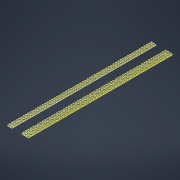
# Autodesk Inventor part: 110033226_ipt_39_背流基座
Saved by Autodesk Inventor 2022 (Build 260153000, 153)
## iProperties
Created: 2022-06-26
Part Number: 110033226_ipt_39_背流基座
Material: 一般
Document SubType Name: Modeling
Designer: User
Density: 1 g/cm^3
Appearance: 預設
Author: User
Autodesk Inventor part; units mm, degrees
ref_plane "YZ Plane" through (0, 0, 0) normal (1, 0, 0) x (0, 1, 0)
ref_plane "XZ Plane" through (0, 0, 0) normal (0, 1, 0) x (-1, 0, 0)
ref_plane "XY Plane" through (0, 0, 0) normal (0, 0, 1) x (1, 0, 0)
sketch "草圖1" plane through (0, 0, 0) normal (0, 1, 0) x (-1, 0, 0)
  line L0 (0, 0) -> (40, 0)
  line L1 (40, 0) -> (40, -305)
  line L2 (40, -305) -> (0, -305)
  line L3 (0, -305) -> (0, 0)
  circle A0 centre (2.5, -2.5) radius 1.7
  line L4 (10, -305) -> (10, 0)
  line L5 (30, -305) -> (30, 0)
  dimension "d0" = 40
  dimension "d1" = 305
  dimension "d2" = 3.4
  dimension "d3" = 2.5
  dimension "d4" = 2.5
  dimension "d45" = 10
  dimension "d46" = 10
  constraints: 12 end point, 4 point on line, 3 perpendicular, 2 parallel, 1 centre point, 1 horizontal
  measures "d0" distance of L1.end L2.end
  measures "d1" distance of L0.end L1.end
  measures "d2" diameter of A0
  measures "d3" distance from line of L3 A0.centre
  measures "d4" distance from line of L0 A0.centre
  measures "d45" distance between parallel lines of L3 L4
  measures "d46" distance between parallel lines of L1 L5
extrude "擠出1" add sketch "草圖1" along normal blind 2.5 contours L0 L4 L2 L3 | L0 L1 L2 L5 | A0
extrude "擠出2" cut sketch "草圖1" along normal blind 1.5 contours A0
sketch "草圖2" plane through (0, 2.5, 0) normal (0, 1, 0) x (1, 0, 0)
  circle A0 centre (-2.5, 2.5) radius 1.7 projected
  point P0 (0, 0)
extrude "擠出3" add sketch "草圖2" along normal blind 1.5
pattern_linear "矩形陣列3" count 61 spacing 5 along (0, 0, -1) count 2 spacing 5 along (-1, 0, 0) of "擠出3", "擠出2"
sketch "草圖3" plane through (0, 2.5, 0) normal (0, 1, 0) x (1, 0, 0)
  circle A0 centre (-2.5, 2.5) radius 1.7 projected
  line L0 (0, 305) -> (0, 0) projected
  line L1 (-30, 0) -> (-40, 0) projected
  line L2 (-40, 0) -> (-40, 305) projected
  line L3 (-40, 305) -> (-30, 305) projected
  circle A1 centre (-2.5, 7.5) radius 1.7 projected
  circle A2 centre (-2.5, 12.5) radius 1.7 projected
  circle A3 centre (-2.5, 17.5) radius 1.7 projected
  circle A4 centre (-2.5, 22.5) radius 1.7 projected
  circle A5 centre (-2.5, 27.5) radius 1.7 projected
  circle A6 centre (-2.5, 32.5) radius 1.7 projected
  circle A7 centre (-2.5, 37.5) radius 1.7 projected
  circle A8 centre (-2.5, 42.5) radius 1.7 projected
  circle A9 centre (-2.5, 47.5) radius 1.7 projected
  circle A10 centre (-2.5, 52.5) radius 1.7 projected
  circle A11 centre (-2.5, 57.5) radius 1.7 projected
  circle A12 centre (-2.5, 62.5) radius 1.7 projected
  circle A13 centre (-2.5, 67.5) radius 1.7 projected
  circle A14 centre (-2.5, 72.5) radius 1.7 projected
  circle A15 centre (-2.5, 77.5) radius 1.7 projected
  circle A16 centre (-2.5, 82.5) radius 1.7 projected
  circle A17 centre (-2.5, 87.5) radius 1.7 projected
  circle A18 centre (-2.5, 92.5) radius 1.7 projected
  circle A19 centre (-2.5, 97.5) radius 1.7 projected
  circle A20 centre (-2.5, 102.5) radius 1.7 projected
  circle A21 centre (-2.5, 107.5) radius 1.7 projected
  circle A22 centre (-2.5, 112.5) radius 1.7 projected
  circle A23 centre (-2.5, 117.5) radius 1.7 projected
  circle A24 centre (-2.5, 122.5) radius 1.7 projected
  circle A25 centre (-2.5, 127.5) radius 1.7 projected
  circle A26 centre (-2.5, 132.5) radius 1.7 projected
  circle A27 centre (-2.5, 137.5) radius 1.7 projected
  circle A28 centre (-2.5, 142.5) radius 1.7 projected
  circle A29 centre (-2.5, 147.5) radius 1.7 projected
  circle A30 centre (-2.5, 152.5) radius 1.7 projected
  circle A31 centre (-2.5, 157.5) radius 1.7 projected
  circle A32 centre (-2.5, 162.5) radius 1.7 projected
  circle A33 centre (-2.5, 167.5) radius 1.7 projected
  circle A34 centre (-2.5, 172.5) radius 1.7 projected
  circle A35 centre (-2.5, 177.5) radius 1.7 projected
  circle A36 centre (-2.5, 182.5) radius 1.7 projected
  circle A37 centre (-2.5, 187.5) radius 1.7 projected
  circle A38 centre (-2.5, 192.5) radius 1.7 projected
  circle A39 centre (-2.5, 197.5) radius 1.7 projected
  circle A40 centre (-2.5, 202.5) radius 1.7 projected
  circle A41 centre (-2.5, 207.5) radius 1.7 projected
  circle A42 centre (-2.5, 212.5) radius 1.7 projected
  circle A43 centre (-2.5, 217.5) radius 1.7 projected
  circle A44 centre (-2.5, 222.5) radius 1.7 projected
  circle A45 centre (-2.5, 227.5) radius 1.7 projected
  circle A46 centre (-2.5, 232.5) radius 1.7 projected
  circle A47 centre (-2.5, 237.5) radius 1.7 projected
  circle A48 centre (-2.5, 242.5) radius 1.7 projected
  circle A49 centre (-2.5, 247.5) radius 1.7 projected
  circle A50 centre (-2.5, 252.5) radius 1.7 projected
  circle A51 centre (-2.5, 257.5) radius 1.7 projected
  circle A52 centre (-2.5, 262.5) radius 1.7 projected
  circle A53 centre (-2.5, 267.5) radius 1.7 projected
  circle A54 centre (-2.5, 272.5) radius 1.7 projected
  circle A55 centre (-2.5, 277.5) radius 1.7 projected
  circle A56 centre (-2.5, 282.5) radius 1.7 projected
  circle A57 centre (-2.5, 287.5) radius 1.7 projected
  circle A58 centre (-2.5, 292.5) radius 1.7 projected
  circle A59 centre (-2.5, 297.5) radius 1.7 projected
  circle A60 centre (-2.5, 302.5) radius 1.7 projected
  circle A61 centre (-7.5, 2.5) radius 1.7 projected
  circle A62 centre (-7.5, 7.5) radius 1.7 projected
  circle A63 centre (-7.5, 12.5) radius 1.7 projected
  circle A64 centre (-7.5, 17.5) radius 1.7 projected
  circle A65 centre (-7.5, 22.5) radius 1.7 projected
  circle A66 centre (-7.5, 27.5) radius 1.7 projected
  circle A67 centre (-7.5, 32.5) radius 1.7 projected
  circle A68 centre (-7.5, 37.5) radius 1.7 projected
  circle A69 centre (-7.5, 42.5) radius 1.7 projected
  circle A70 centre (-7.5, 47.5) radius 1.7 projected
  circle A71 centre (-7.5, 52.5) radius 1.7 projected
  circle A72 centre (-7.5, 57.5) radius 1.7 projected
  circle A73 centre (-7.5, 62.5) radius 1.7 projected
  circle A74 centre (-7.5, 67.5) radius 1.7 projected
  circle A75 centre (-7.5, 72.5) radius 1.7 projected
  circle A76 centre (-7.5, 77.5) radius 1.7 projected
  circle A77 centre (-7.5, 82.5) radius 1.7 projected
  circle A78 centre (-7.5, 87.5) radius 1.7 projected
  circle A79 centre (-7.5, 92.5) radius 1.7 projected
  circle A80 centre (-7.5, 97.5) radius 1.7 projected
  circle A81 centre (-7.5, 102.5) radius 1.7 projected
  circle A82 centre (-7.5, 107.5) radius 1.7 projected
  circle A83 centre (-7.5, 112.5) radius 1.7 projected
  circle A84 centre (-7.5, 117.5) radius 1.7 projected
  circle A85 centre (-7.5, 122.5) radius 1.7 projected
  circle A86 centre (-7.5, 127.5) radius 1.7 projected
  circle A87 centre (-7.5, 132.5) radius 1.7 projected
  circle A88 centre (-7.5, 137.5) radius 1.7 projected
  circle A89 centre (-7.5, 142.5) radius 1.7 projected
  circle A90 centre (-7.5, 147.5) radius 1.7 projected
  circle A91 centre (-7.5, 152.5) radius 1.7 projected
  circle A92 centre (-7.5, 157.5) radius 1.7 projected
  circle A93 centre (-7.5, 162.5) radius 1.7 projected
  circle A94 centre (-7.5, 167.5) radius 1.7 projected
  circle A95 centre (-7.5, 172.5) radius 1.7 projected
  circle A96 centre (-7.5, 177.5) radius 1.7 projected
  circle A97 centre (-7.5, 182.5) radius 1.7 projected
  circle A98 centre (-7.5, 187.5) radius 1.7 projected
  circle A99 centre (-7.5, 192.5) radius 1.7 projected
  circle A100 centre (-7.5, 197.5) radius 1.7 projected
  circle A101 centre (-7.5, 202.5) radius 1.7 projected
  circle A102 centre (-7.5, 207.5) radius 1.7 projected
  circle A103 centre (-7.5, 212.5) radius 1.7 projected
  circle A104 centre (-7.5, 217.5) radius 1.7 projected
  circle A105 centre (-7.5, 222.5) radius 1.7 projected
  circle A106 centre (-7.5, 227.5) radius 1.7 projected
  circle A107 centre (-7.5, 232.5) radius 1.7 projected
  circle A108 centre (-7.5, 237.5) radius 1.7 projected
  circle A109 centre (-7.5, 242.5) radius 1.7 projected
  circle A110 centre (-7.5, 247.5) radius 1.7 projected
  circle A111 centre (-7.5, 252.5) radius 1.7 projected
  circle A112 centre (-7.5, 257.5) radius 1.7 projected
  circle A113 centre (-7.5, 262.5) radius 1.7 projected
  circle A114 centre (-7.5, 267.5) radius 1.7 projected
  circle A115 centre (-7.5, 272.5) radius 1.7 projected
  circle A116 centre (-7.5, 277.5) radius 1.7 projected
  circle A117 centre (-7.5, 282.5) radius 1.7 projected
  circle A118 centre (-7.5, 287.5) radius 1.7 projected
  circle A119 centre (-7.5, 292.5) radius 1.7 projected
  circle A120 centre (-7.5, 297.5) radius 1.7 projected
  circle A121 centre (-7.5, 302.5) radius 1.7 projected
  circle A122 centre (-37.5, 2.5) radius 1.7
  line L4 (-30, 305) -> (-30, 0) projected
  line L5 (0, 0) -> (-10, 0) projected
  line L6 (-10, 0) -> (-10, 305) projected
  line L7 (-10, 305) -> (0, 305) projected
  dimension "d26" = 3.4
  dimension "d27" = 2.5
  dimension "d28" = 2.5
  constraints: 1 centre point
  measures "d26" diameter of A122
  measures "d27" distance from line of L2 A122.centre
  measures "d28" distance from line of L1 A122.centre
extrude "擠出4" add sketch "草圖3" along normal blind 1.5 contours A122
pattern_linear "矩形陣列4" count 61 spacing 5 along (0, 0, -1) count 2 spacing 5 along (1, 0, 0) of "擠出4"
sketch "草圖4" plane through (0, 0, 0) normal (0, -1, 0) x (1, 0, 0)
  circle A0 centre (-37.5, -2.5) radius 1.7 projected
  point P0 (0, 0)
extrude "擠出5" cut sketch "草圖4" against normal blind 1.5
pattern_linear "矩形陣列5" count 2 spacing 5 along (1, 0, 0) count 61 spacing 5 along (0, 0, -1) of "擠出5"
sketch "草圖5" plane through (0, 0, 0) normal (1, 0, 0) x (0, 0, -1)
  line L0 (305, 2.5) -> (305, 0) projected
  line L1 (305, 0) -> (0, 0) projected
  line L2 (0, 0) -> (0, 2.5) projected
  line L3 (0, 2.5) -> (305, 2.5) projected
extrude "擠出6" add sketch "草圖5" along normal blind 5
sketch "草圖6" plane through (0, 2.5, 0) normal (0, 1, 0) x (1, 0, 0)
  line L0 (5, 305) -> (5, 0) projected
  line L1 (5, 0) -> (-10, 0) projected
  line L2 (-10, 0) -> (-10, 305) projected
  line L3 (-10, 305) -> (5, 305) projected
  circle A0 centre (-2.5, 2.5) radius 1.7 projected
  circle A1 centre (-2.5, 7.5) radius 1.7 projected
  circle A2 centre (-2.5, 12.5) radius 1.7 projected
  circle A3 centre (-2.5, 17.5) radius 1.7 projected
  circle A4 centre (-2.5, 22.5) radius 1.7 projected
  circle A5 centre (-2.5, 27.5) radius 1.7 projected
  circle A6 centre (-2.5, 32.5) radius 1.7 projected
  circle A7 centre (-2.5, 37.5) radius 1.7 projected
  circle A8 centre (-2.5, 42.5) radius 1.7 projected
  circle A9 centre (-2.5, 47.5) radius 1.7 projected
  circle A10 centre (-2.5, 52.5) radius 1.7 projected
  circle A11 centre (-2.5, 57.5) radius 1.7 projected
  circle A12 centre (-2.5, 62.5) radius 1.7 projected
  circle A13 centre (-2.5, 67.5) radius 1.7 projected
  circle A14 centre (-2.5, 72.5) radius 1.7 projected
  circle A15 centre (-2.5, 77.5) radius 1.7 projected
  circle A16 centre (-2.5, 82.5) radius 1.7 projected
  circle A17 centre (-2.5, 87.5) radius 1.7 projected
  circle A18 centre (-2.5, 92.5) radius 1.7 projected
  circle A19 centre (-2.5, 97.5) radius 1.7 projected
  circle A20 centre (-2.5, 102.5) radius 1.7 projected
  circle A21 centre (-2.5, 107.5) radius 1.7 projected
  circle A22 centre (-2.5, 112.5) radius 1.7 projected
  circle A23 centre (-2.5, 117.5) radius 1.7 projected
  circle A24 centre (-2.5, 122.5) radius 1.7 projected
  circle A25 centre (-2.5, 127.5) radius 1.7 projected
  circle A26 centre (-2.5, 132.5) radius 1.7 projected
  circle A27 centre (-2.5, 137.5) radius 1.7 projected
  circle A28 centre (-2.5, 142.5) radius 1.7 projected
  circle A29 centre (-2.5, 147.5) radius 1.7 projected
  circle A30 centre (-2.5, 152.5) radius 1.7 projected
  circle A31 centre (-2.5, 157.5) radius 1.7 projected
  circle A32 centre (-2.5, 162.5) radius 1.7 projected
  circle A33 centre (-2.5, 167.5) radius 1.7 projected
  circle A34 centre (-2.5, 172.5) radius 1.7 projected
  circle A35 centre (-2.5, 177.5) radius 1.7 projected
  circle A36 centre (-2.5, 182.5) radius 1.7 projected
  circle A37 centre (-2.5, 187.5) radius 1.7 projected
  circle A38 centre (-2.5, 192.5) radius 1.7 projected
  circle A39 centre (-2.5, 197.5) radius 1.7 projected
  circle A40 centre (-2.5, 202.5) radius 1.7 projected
  circle A41 centre (-2.5, 207.5) radius 1.7 projected
  circle A42 centre (-2.5, 212.5) radius 1.7 projected
  circle A43 centre (-2.5, 217.5) radius 1.7 projected
  circle A44 centre (-2.5, 222.5) radius 1.7 projected
  circle A45 centre (-2.5, 227.5) radius 1.7 projected
  circle A46 centre (-2.5, 232.5) radius 1.7 projected
  circle A47 centre (-2.5, 237.5) radius 1.7 projected
  circle A48 centre (-2.5, 242.5) radius 1.7 projected
  circle A49 centre (-2.5, 247.5) radius 1.7 projected
  circle A50 centre (-2.5, 252.5) radius 1.7 projected
  circle A51 centre (-2.5, 257.5) radius 1.7 projected
  circle A52 centre (-2.5, 262.5) radius 1.7 projected
  circle A53 centre (-2.5, 267.5) radius 1.7 projected
  circle A54 centre (-2.5, 272.5) radius 1.7 projected
  circle A55 centre (-2.5, 277.5) radius 1.7 projected
  circle A56 centre (-2.5, 282.5) radius 1.7 projected
  circle A57 centre (-2.5, 287.5) radius 1.7 projected
  circle A58 centre (-2.5, 292.5) radius 1.7 projected
  circle A59 centre (-2.5, 297.5) radius 1.7 projected
  circle A60 centre (-2.5, 302.5) radius 1.7 projected
  circle A61 centre (-7.5, 2.5) radius 1.7 projected
  circle A62 centre (-7.5, 7.5) radius 1.7 projected
  circle A63 centre (-7.5, 12.5) radius 1.7 projected
  circle A64 centre (-7.5, 17.5) radius 1.7 projected
  circle A65 centre (-7.5, 22.5) radius 1.7 projected
  circle A66 centre (-7.5, 27.5) radius 1.7 projected
  circle A67 centre (-7.5, 32.5) radius 1.7 projected
  circle A68 centre (-7.5, 37.5) radius 1.7 projected
  circle A69 centre (-7.5, 42.5) radius 1.7 projected
  circle A70 centre (-7.5, 47.5) radius 1.7 projected
  circle A71 centre (-7.5, 52.5) radius 1.7 projected
  circle A72 centre (-7.5, 57.5) radius 1.7 projected
  circle A73 centre (-7.5, 62.5) radius 1.7 projected
  circle A74 centre (-7.5, 67.5) radius 1.7 projected
  circle A75 centre (-7.5, 72.5) radius 1.7 projected
  circle A76 centre (-7.5, 77.5) radius 1.7 projected
  circle A77 centre (-7.5, 82.5) radius 1.7 projected
  circle A78 centre (-7.5, 87.5) radius 1.7 projected
  circle A79 centre (-7.5, 92.5) radius 1.7 projected
  circle A80 centre (-7.5, 97.5) radius 1.7 projected
  circle A81 centre (-7.5, 102.5) radius 1.7 projected
  circle A82 centre (-7.5, 107.5) radius 1.7 projected
  circle A83 centre (-7.5, 112.5) radius 1.7 projected
  circle A84 centre (-7.5, 117.5) radius 1.7 projected
  circle A85 centre (-7.5, 122.5) radius 1.7 projected
  circle A86 centre (-7.5, 127.5) radius 1.7 projected
  circle A87 centre (-7.5, 132.5) radius 1.7 projected
  circle A88 centre (-7.5, 137.5) radius 1.7 projected
  circle A89 centre (-7.5, 142.5) radius 1.7 projected
  circle A90 centre (-7.5, 147.5) radius 1.7 projected
  circle A91 centre (-7.5, 152.5) radius 1.7 projected
  circle A92 centre (-7.5, 157.5) radius 1.7 projected
  circle A93 centre (-7.5, 162.5) radius 1.7 projected
  circle A94 centre (-7.5, 167.5) radius 1.7 projected
  circle A95 centre (-7.5, 172.5) radius 1.7 projected
  circle A96 centre (-7.5, 177.5) radius 1.7 projected
  circle A97 centre (-7.5, 182.5) radius 1.7 projected
  circle A98 centre (-7.5, 187.5) radius 1.7 projected
  circle A99 centre (-7.5, 192.5) radius 1.7 projected
  circle A100 centre (-7.5, 197.5) radius 1.7 projected
  circle A101 centre (-7.5, 202.5) radius 1.7 projected
  circle A102 centre (-7.5, 207.5) radius 1.7 projected
  circle A103 centre (-7.5, 212.5) radius 1.7 projected
  circle A104 centre (-7.5, 217.5) radius 1.7 projected
  circle A105 centre (-7.5, 222.5) radius 1.7 projected
  circle A106 centre (-7.5, 227.5) radius 1.7 projected
  circle A107 centre (-7.5, 232.5) radius 1.7 projected
  circle A108 centre (-7.5, 237.5) radius 1.7 projected
  circle A109 centre (-7.5, 242.5) radius 1.7 projected
  circle A110 centre (-7.5, 247.5) radius 1.7 projected
  circle A111 centre (-7.5, 252.5) radius 1.7 projected
  circle A112 centre (-7.5, 257.5) radius 1.7 projected
  circle A113 centre (-7.5, 262.5) radius 1.7 projected
  circle A114 centre (-7.5, 267.5) radius 1.7 projected
  circle A115 centre (-7.5, 272.5) radius 1.7 projected
  circle A116 centre (-7.5, 277.5) radius 1.7 projected
  circle A117 centre (-7.5, 282.5) radius 1.7 projected
  circle A118 centre (-7.5, 287.5) radius 1.7 projected
  circle A119 centre (-7.5, 292.5) radius 1.7 projected
  circle A120 centre (-7.5, 297.5) radius 1.7 projected
  circle A121 centre (-7.5, 302.5) radius 1.7 projected
  circle A122 centre (-37.5, 2.5) radius 1.7 projected
  line L4 (-40, 0) -> (-40, 305) projected
  line L5 (-40, 305) -> (-30, 305) projected
  line L6 (-30, 305) -> (-30, 0) projected
  line L7 (-30, 0) -> (-40, 0) projected
  circle A123 centre (-37.5, 7.5) radius 1.7 projected
  circle A124 centre (-37.5, 12.5) radius 1.7 projected
  circle A125 centre (-37.5, 17.5) radius 1.7 projected
  circle A126 centre (-37.5, 22.5) radius 1.7 projected
  circle A127 centre (-37.5, 27.5) radius 1.7 projected
  circle A128 centre (-37.5, 32.5) radius 1.7 projected
  circle A129 centre (-37.5, 37.5) radius 1.7 projected
  circle A130 centre (-37.5, 42.5) radius 1.7 projected
  circle A131 centre (-37.5, 47.5) radius 1.7 projected
  circle A132 centre (-37.5, 52.5) radius 1.7 projected
  circle A133 centre (-37.5, 57.5) radius 1.7 projected
  circle A134 centre (-37.5, 62.5) radius 1.7 projected
  circle A135 centre (-37.5, 67.5) radius 1.7 projected
  circle A136 centre (-37.5, 72.5) radius 1.7 projected
  circle A137 centre (-37.5, 77.5) radius 1.7 projected
  circle A138 centre (-37.5, 82.5) radius 1.7 projected
  circle A139 centre (-37.5, 87.5) radius 1.7 projected
  circle A140 centre (-37.5, 92.5) radius 1.7 projected
  circle A141 centre (-37.5, 97.5) radius 1.7 projected
  circle A142 centre (-37.5, 102.5) radius 1.7 projected
  circle A143 centre (-37.5, 107.5) radius 1.7 projected
  circle A144 centre (-37.5, 112.5) radius 1.7 projected
  circle A145 centre (-37.5, 117.5) radius 1.7 projected
  circle A146 centre (-37.5, 122.5) radius 1.7 projected
  circle A147 centre (-37.5, 127.5) radius 1.7 projected
  circle A148 centre (-37.5, 132.5) radius 1.7 projected
  circle A149 centre (-37.5, 137.5) radius 1.7 projected
  circle A150 centre (-37.5, 142.5) radius 1.7 projected
  circle A151 centre (-37.5, 147.5) radius 1.7 projected
  circle A152 centre (-37.5, 152.5) radius 1.7 projected
  circle A153 centre (-37.5, 157.5) radius 1.7 projected
  circle A154 centre (-37.5, 162.5) radius 1.7 projected
  circle A155 centre (-37.5, 167.5) radius 1.7 projected
  circle A156 centre (-37.5, 172.5) radius 1.7 projected
  circle A157 centre (-37.5, 177.5) radius 1.7 projected
  circle A158 centre (-37.5, 182.5) radius 1.7 projected
  circle A159 centre (-37.5, 187.5) radius 1.7 projected
  circle A160 centre (-37.5, 192.5) radius 1.7 projected
  circle A161 centre (-37.5, 197.5) radius 1.7 projected
  circle A162 centre (-37.5, 202.5) radius 1.7 projected
  circle A163 centre (-37.5, 207.5) radius 1.7 projected
  circle A164 centre (-37.5, 212.5) radius 1.7 projected
  circle A165 centre (-37.5, 217.5) radius 1.7 projected
  circle A166 centre (-37.5, 222.5) radius 1.7 projected
  circle A167 centre (-37.5, 227.5) radius 1.7 projected
  circle A168 centre (-37.5, 232.5) radius 1.7 projected
  circle A169 centre (-37.5, 237.5) radius 1.7 projected
  circle A170 centre (-37.5, 242.5) radius 1.7 projected
  circle A171 centre (-37.5, 247.5) radius 1.7 projected
  circle A172 centre (-37.5, 252.5) radius 1.7 projected
  circle A173 centre (-37.5, 257.5) radius 1.7 projected
  circle A174 centre (-37.5, 262.5) radius 1.7 projected
  circle A175 centre (-37.5, 267.5) radius 1.7 projected
  circle A176 centre (-37.5, 272.5) radius 1.7 projected
  circle A177 centre (-37.5, 277.5) radius 1.7 projected
  circle A178 centre (-37.5, 282.5) radius 1.7 projected
  circle A179 centre (-37.5, 287.5) radius 1.7 projected
  circle A180 centre (-37.5, 292.5) radius 1.7 projected
  circle A181 centre (-37.5, 297.5) radius 1.7 projected
  circle A182 centre (-37.5, 302.5) radius 1.7 projected
  circle A183 centre (-32.5, 2.5) radius 1.7 projected
  circle A184 centre (-32.5, 7.5) radius 1.7 projected
  circle A185 centre (-32.5, 12.5) radius 1.7 projected
  circle A186 centre (-32.5, 17.5) radius 1.7 projected
  circle A187 centre (-32.5, 22.5) radius 1.7 projected
  circle A188 centre (-32.5, 27.5) radius 1.7 projected
  circle A189 centre (-32.5, 32.5) radius 1.7 projected
  circle A190 centre (-32.5, 37.5) radius 1.7 projected
  circle A191 centre (-32.5, 42.5) radius 1.7 projected
  circle A192 centre (-32.5, 47.5) radius 1.7 projected
  circle A193 centre (-32.5, 52.5) radius 1.7 projected
  circle A194 centre (-32.5, 57.5) radius 1.7 projected
  circle A195 centre (-32.5, 62.5) radius 1.7 projected
  circle A196 centre (-32.5, 67.5) radius 1.7 projected
  circle A197 centre (-32.5, 72.5) radius 1.7 projected
  circle A198 centre (-32.5, 77.5) radius 1.7 projected
  circle A199 centre (-32.5, 82.5) radius 1.7 projected
  circle A200 centre (-32.5, 87.5) radius 1.7 projected
  circle A201 centre (-32.5, 92.5) radius 1.7 projected
  circle A202 centre (-32.5, 97.5) radius 1.7 projected
  circle A203 centre (-32.5, 102.5) radius 1.7 projected
  circle A204 centre (-32.5, 107.5) radius 1.7 projected
  circle A205 centre (-32.5, 112.5) radius 1.7 projected
  circle A206 centre (-32.5, 117.5) radius 1.7 projected
  circle A207 centre (-32.5, 122.5) radius 1.7 projected
  circle A208 centre (-32.5, 127.5) radius 1.7 projected
  circle A209 centre (-32.5, 132.5) radius 1.7 projected
  circle A210 centre (-32.5, 137.5) radius 1.7 projected
  circle A211 centre (-32.5, 142.5) radius 1.7 projected
  circle A212 centre (-32.5, 147.5) radius 1.7 projected
  circle A213 centre (-32.5, 152.5) radius 1.7 projected
  circle A214 centre (-32.5, 157.5) radius 1.7 projected
  circle A215 centre (-32.5, 162.5) radius 1.7 projected
  circle A216 centre (-32.5, 167.5) radius 1.7 projected
  circle A217 centre (-32.5, 172.5) radius 1.7 projected
  circle A218 centre (-32.5, 177.5) radius 1.7 projected
  circle A219 centre (-32.5, 182.5) radius 1.7 projected
  circle A220 centre (-32.5, 187.5) radius 1.7 projected
  circle A221 centre (-32.5, 192.5) radius 1.7 projected
  circle A222 centre (-32.5, 197.5) radius 1.7 projected
  circle A223 centre (-32.5, 202.5) radius 1.7 projected
  circle A224 centre (-32.5, 207.5) radius 1.7 projected
  circle A225 centre (-32.5, 212.5) radius 1.7 projected
  circle A226 centre (-32.5, 217.5) radius 1.7 projected
  circle A227 centre (-32.5, 222.5) radius 1.7 projected
  circle A228 centre (-32.5, 227.5) radius 1.7 projected
  circle A229 centre (-32.5, 232.5) radius 1.7 projected
  circle A230 centre (-32.5, 237.5) radius 1.7 projected
  circle A231 centre (-32.5, 242.5) radius 1.7 projected
  circle A232 centre (-32.5, 247.5) radius 1.7 projected
  circle A233 centre (-32.5, 252.5) radius 1.7 projected
  circle A234 centre (-32.5, 257.5) radius 1.7 projected
  circle A235 centre (-32.5, 262.5) radius 1.7 projected
  circle A236 centre (-32.5, 267.5) radius 1.7 projected
  circle A237 centre (-32.5, 272.5) radius 1.7 projected
  circle A238 centre (-32.5, 277.5) radius 1.7 projected
  circle A239 centre (-32.5, 282.5) radius 1.7 projected
  circle A240 centre (-32.5, 287.5) radius 1.7 projected
  circle A241 centre (-32.5, 292.5) radius 1.7 projected
  circle A242 centre (-32.5, 297.5) radius 1.7 projected
  circle A243 centre (-32.5, 302.5) radius 1.7 projected
  circle A244 centre (2.5, 2.5) radius 1.7
  point P0 (0, 0)
  dimension "d49" = 3.4
  dimension "d50" = 2.5
  dimension "d51" = 2.5
  constraints: 1 centre point
  measures "d49" diameter of A244
  measures "d50" distance from line of L0 A244.centre
  measures "d51" distance from line of L1 A244.centre
extrude "擠出7" add sketch "草圖6" along normal blind 1.5 contours A244
sketch "草圖7" plane through (0, 0, 0) normal (0, -1, 0) x (1, 0, 0)
  circle A0 centre (-37.5, -2.5) radius 1.7 projected
  line L0 (-40, -305) -> (-40, 0) projected
  line L1 (-40, 0) -> (-30, 0) projected
  line L2 (-30, 0) -> (-30, -305) projected
  line L3 (-30, -305) -> (-40, -305) projected
  circle A1 centre (-32.5, -2.5) radius 1.7 projected
  circle A2 centre (-37.5, -7.5) radius 1.7 projected
  circle A3 centre (-32.5, -7.5) radius 1.7 projected
  circle A4 centre (-37.5, -12.5) radius 1.7 projected
  circle A5 centre (-32.5, -12.5) radius 1.7 projected
  circle A6 centre (-37.5, -17.5) radius 1.7 projected
  circle A7 centre (-32.5, -17.5) radius 1.7 projected
  circle A8 centre (-37.5, -22.5) radius 1.7 projected
  circle A9 centre (-32.5, -22.5) radius 1.7 projected
  circle A10 centre (-37.5, -27.5) radius 1.7 projected
  circle A11 centre (-32.5, -27.5) radius 1.7 projected
  circle A12 centre (-37.5, -32.5) radius 1.7 projected
  circle A13 centre (-32.5, -32.5) radius 1.7 projected
  circle A14 centre (-37.5, -37.5) radius 1.7 projected
  circle A15 centre (-32.5, -37.5) radius 1.7 projected
  circle A16 centre (-37.5, -42.5) radius 1.7 projected
  circle A17 centre (-32.5, -42.5) radius 1.7 projected
  circle A18 centre (-37.5, -47.5) radius 1.7 projected
  circle A19 centre (-32.5, -47.5) radius 1.7 projected
  circle A20 centre (-37.5, -52.5) radius 1.7 projected
  circle A21 centre (-32.5, -52.5) radius 1.7 projected
  circle A22 centre (-37.5, -57.5) radius 1.7 projected
  circle A23 centre (-32.5, -57.5) radius 1.7 projected
  circle A24 centre (-37.5, -62.5) radius 1.7 projected
  circle A25 centre (-32.5, -62.5) radius 1.7 projected
  circle A26 centre (-37.5, -67.5) radius 1.7 projected
  circle A27 centre (-32.5, -67.5) radius 1.7 projected
  circle A28 centre (-37.5, -72.5) radius 1.7 projected
  circle A29 centre (-32.5, -72.5) radius 1.7 projected
  circle A30 centre (-37.5, -77.5) radius 1.7 projected
  circle A31 centre (-32.5, -77.5) radius 1.7 projected
  circle A32 centre (-37.5, -82.5) radius 1.7 projected
  circle A33 centre (-32.5, -82.5) radius 1.7 projected
  circle A34 centre (-37.5, -87.5) radius 1.7 projected
  circle A35 centre (-32.5, -87.5) radius 1.7 projected
  circle A36 centre (-37.5, -92.5) radius 1.7 projected
  circle A37 centre (-32.5, -92.5) radius 1.7 projected
  circle A38 centre (-37.5, -97.5) radius 1.7 projected
  circle A39 centre (-32.5, -97.5) radius 1.7 projected
  circle A40 centre (-37.5, -102.5) radius 1.7 projected
  circle A41 centre (-32.5, -102.5) radius 1.7 projected
  circle A42 centre (-37.5, -107.5) radius 1.7 projected
  circle A43 centre (-32.5, -107.5) radius 1.7 projected
  circle A44 centre (-37.5, -112.5) radius 1.7 projected
  circle A45 centre (-32.5, -112.5) radius 1.7 projected
  circle A46 centre (-37.5, -117.5) radius 1.7 projected
  circle A47 centre (-32.5, -117.5) radius 1.7 projected
  circle A48 centre (-37.5, -122.5) radius 1.7 projected
  circle A49 centre (-32.5, -122.5) radius 1.7 projected
  circle A50 centre (-37.5, -127.5) radius 1.7 projected
  circle A51 centre (-32.5, -127.5) radius 1.7 projected
  circle A52 centre (-37.5, -132.5) radius 1.7 projected
  circle A53 centre (-32.5, -132.5) radius 1.7 projected
  circle A54 centre (-37.5, -137.5) radius 1.7 projected
  circle A55 centre (-32.5, -137.5) radius 1.7 projected
  circle A56 centre (-37.5, -142.5) radius 1.7 projected
  circle A57 centre (-32.5, -142.5) radius 1.7 projected
  circle A58 centre (-37.5, -147.5) radius 1.7 projected
  circle A59 centre (-32.5, -147.5) radius 1.7 projected
  circle A60 centre (-37.5, -152.5) radius 1.7 projected
  circle A61 centre (-32.5, -152.5) radius 1.7 projected
  circle A62 centre (-37.5, -157.5) radius 1.7 projected
  circle A63 centre (-32.5, -157.5) radius 1.7 projected
  circle A64 centre (-37.5, -162.5) radius 1.7 projected
  circle A65 centre (-32.5, -162.5) radius 1.7 projected
  circle A66 centre (-37.5, -167.5) radius 1.7 projected
  circle A67 centre (-32.5, -167.5) radius 1.7 projected
  circle A68 centre (-37.5, -172.5) radius 1.7 projected
  circle A69 centre (-32.5, -172.5) radius 1.7 projected
  circle A70 centre (-37.5, -177.5) radius 1.7 projected
  circle A71 centre (-32.5, -177.5) radius 1.7 projected
  circle A72 centre (-37.5, -182.5) radius 1.7 projected
  circle A73 centre (-32.5, -182.5) radius 1.7 projected
  circle A74 centre (-37.5, -187.5) radius 1.7 projected
  circle A75 centre (-32.5, -187.5) radius 1.7 projected
  circle A76 centre (-37.5, -192.5) radius 1.7 projected
  circle A77 centre (-32.5, -192.5) radius 1.7 projected
  circle A78 centre (-37.5, -197.5) radius 1.7 projected
  circle A79 centre (-32.5, -197.5) radius 1.7 projected
  circle A80 centre (-37.5, -202.5) radius 1.7 projected
  circle A81 centre (-32.5, -202.5) radius 1.7 projected
  circle A82 centre (-37.5, -207.5) radius 1.7 projected
  circle A83 centre (-32.5, -207.5) radius 1.7 projected
  circle A84 centre (-37.5, -212.5) radius 1.7 projected
  circle A85 centre (-32.5, -212.5) radius 1.7 projected
  circle A86 centre (-37.5, -217.5) radius 1.7 projected
  circle A87 centre (-32.5, -217.5) radius 1.7 projected
  circle A88 centre (-37.5, -222.5) radius 1.7 projected
  circle A89 centre (-32.5, -222.5) radius 1.7 projected
  circle A90 centre (-37.5, -227.5) radius 1.7 projected
  circle A91 centre (-32.5, -227.5) radius 1.7 projected
  circle A92 centre (-37.5, -232.5) radius 1.7 projected
  circle A93 centre (-32.5, -232.5) radius 1.7 projected
  circle A94 centre (-37.5, -237.5) radius 1.7 projected
  circle A95 centre (-32.5, -237.5) radius 1.7 projected
  circle A96 centre (-37.5, -242.5) radius 1.7 projected
  circle A97 centre (-32.5, -242.5) radius 1.7 projected
  circle A98 centre (-37.5, -247.5) radius 1.7 projected
  circle A99 centre (-32.5, -247.5) radius 1.7 projected
  circle A100 centre (-37.5, -252.5) radius 1.7 projected
  circle A101 centre (-32.5, -252.5) radius 1.7 projected
  circle A102 centre (-37.5, -257.5) radius 1.7 projected
  circle A103 centre (-32.5, -257.5) radius 1.7 projected
  circle A104 centre (-37.5, -262.5) radius 1.7 projected
  circle A105 centre (-32.5, -262.5) radius 1.7 projected
  circle A106 centre (-37.5, -267.5) radius 1.7 projected
  circle A107 centre (-32.5, -267.5) radius 1.7 projected
  circle A108 centre (-37.5, -272.5) radius 1.7 projected
  circle A109 centre (-32.5, -272.5) radius 1.7 projected
  circle A110 centre (-37.5, -277.5) radius 1.7 projected
  circle A111 centre (-32.5, -277.5) radius 1.7 projected
  circle A112 centre (-37.5, -282.5) radius 1.7 projected
  circle A113 centre (-32.5, -282.5) radius 1.7 projected
  circle A114 centre (-37.5, -287.5) radius 1.7 projected
  circle A115 centre (-32.5, -287.5) radius 1.7 projected
  circle A116 centre (-37.5, -292.5) radius 1.7 projected
  circle A117 centre (-32.5, -292.5) radius 1.7 projected
  circle A118 centre (-37.5, -297.5) radius 1.7 projected
  circle A119 centre (-32.5, -297.5) radius 1.7 projected
  circle A120 centre (-37.5, -302.5) radius 1.7 projected
  circle A121 centre (-32.5, -302.5) radius 1.7 projected
  line L4 (5, 0) -> (5, -305) projected
  line L5 (5, -305) -> (-10, -305) projected
  line L6 (-10, -305) -> (-10, 0) projected
  line L7 (-10, 0) -> (5, 0) projected
  circle A122 centre (-2.5, -2.5) radius 1.7 projected
  circle A123 centre (-2.5, -7.5) radius 1.7 projected
  circle A124 centre (-2.5, -12.5) radius 1.7 projected
  circle A125 centre (-2.5, -17.5) radius 1.7 projected
  circle A126 centre (-2.5, -22.5) radius 1.7 projected
  circle A127 centre (-2.5, -27.5) radius 1.7 projected
  circle A128 centre (-2.5, -32.5) radius 1.7 projected
  circle A129 centre (-2.5, -37.5) radius 1.7 projected
  circle A130 centre (-2.5, -42.5) radius 1.7 projected
  circle A131 centre (-2.5, -47.5) radius 1.7 projected
  circle A132 centre (-2.5, -52.5) radius 1.7 projected
  circle A133 centre (-2.5, -57.5) radius 1.7 projected
  circle A134 centre (-2.5, -62.5) radius 1.7 projected
  circle A135 centre (-2.5, -67.5) radius 1.7 projected
  circle A136 centre (-2.5, -72.5) radius 1.7 projected
  circle A137 centre (-2.5, -77.5) radius 1.7 projected
  circle A138 centre (-2.5, -82.5) radius 1.7 projected
  circle A139 centre (-2.5, -87.5) radius 1.7 projected
  circle A140 centre (-2.5, -92.5) radius 1.7 projected
  circle A141 centre (-2.5, -97.5) radius 1.7 projected
  circle A142 centre (-2.5, -102.5) radius 1.7 projected
  circle A143 centre (-2.5, -107.5) radius 1.7 projected
  circle A144 centre (-2.5, -112.5) radius 1.7 projected
  circle A145 centre (-2.5, -117.5) radius 1.7 projected
  circle A146 centre (-2.5, -122.5) radius 1.7 projected
  circle A147 centre (-2.5, -127.5) radius 1.7 projected
  circle A148 centre (-2.5, -132.5) radius 1.7 projected
  circle A149 centre (-2.5, -137.5) radius 1.7 projected
  circle A150 centre (-2.5, -142.5) radius 1.7 projected
  circle A151 centre (-2.5, -147.5) radius 1.7 projected
  circle A152 centre (-2.5, -152.5) radius 1.7 projected
  circle A153 centre (-2.5, -157.5) radius 1.7 projected
  circle A154 centre (-2.5, -162.5) radius 1.7 projected
  circle A155 centre (-2.5, -167.5) radius 1.7 projected
  circle A156 centre (-2.5, -172.5) radius 1.7 projected
  circle A157 centre (-2.5, -177.5) radius 1.7 projected
  circle A158 centre (-2.5, -182.5) radius 1.7 projected
  circle A159 centre (-2.5, -187.5) radius 1.7 projected
  circle A160 centre (-2.5, -192.5) radius 1.7 projected
  circle A161 centre (-2.5, -197.5) radius 1.7 projected
  circle A162 centre (-2.5, -202.5) radius 1.7 projected
  circle A163 centre (-2.5, -207.5) radius 1.7 projected
  circle A164 centre (-2.5, -212.5) radius 1.7 projected
  circle A165 centre (-2.5, -217.5) radius 1.7 projected
  circle A166 centre (-2.5, -222.5) radius 1.7 projected
  circle A167 centre (-2.5, -227.5) radius 1.7 projected
  circle A168 centre (-2.5, -232.5) radius 1.7 projected
  circle A169 centre (-2.5, -237.5) radius 1.7 projected
  circle A170 centre (-2.5, -242.5) radius 1.7 projected
  circle A171 centre (-2.5, -247.5) radius 1.7 projected
  circle A172 centre (-2.5, -252.5) radius 1.7 projected
  circle A173 centre (-2.5, -257.5) radius 1.7 projected
  circle A174 centre (-2.5, -262.5) radius 1.7 projected
  circle A175 centre (-2.5, -267.5) radius 1.7 projected
  circle A176 centre (-2.5, -272.5) radius 1.7 projected
  circle A177 centre (-2.5, -277.5) radius 1.7 projected
  circle A178 centre (-2.5, -282.5) radius 1.7 projected
  circle A179 centre (-2.5, -287.5) radius 1.7 projected
  circle A180 centre (-2.5, -292.5) radius 1.7 projected
  circle A181 centre (-2.5, -297.5) radius 1.7 projected
  circle A182 centre (-2.5, -302.5) radius 1.7 projected
  circle A183 centre (-7.5, -2.5) radius 1.7 projected
  circle A184 centre (-7.5, -7.5) radius 1.7 projected
  circle A185 centre (-7.5, -12.5) radius 1.7 projected
  circle A186 centre (-7.5, -17.5) radius 1.7 projected
  circle A187 centre (-7.5, -22.5) radius 1.7 projected
  circle A188 centre (-7.5, -27.5) radius 1.7 projected
  circle A189 centre (-7.5, -32.5) radius 1.7 projected
  circle A190 centre (-7.5, -37.5) radius 1.7 projected
  circle A191 centre (-7.5, -42.5) radius 1.7 projected
  circle A192 centre (-7.5, -47.5) radius 1.7 projected
  circle A193 centre (-7.5, -52.5) radius 1.7 projected
  circle A194 centre (-7.5, -57.5) radius 1.7 projected
  circle A195 centre (-7.5, -62.5) radius 1.7 projected
  circle A196 centre (-7.5, -67.5) radius 1.7 projected
  circle A197 centre (-7.5, -72.5) radius 1.7 projected
  circle A198 centre (-7.5, -77.5) radius 1.7 projected
  circle A199 centre (-7.5, -82.5) radius 1.7 projected
  circle A200 centre (-7.5, -87.5) radius 1.7 projected
  circle A201 centre (-7.5, -92.5) radius 1.7 projected
  circle A202 centre (-7.5, -97.5) radius 1.7 projected
  circle A203 centre (-7.5, -102.5) radius 1.7 projected
  circle A204 centre (-7.5, -107.5) radius 1.7 projected
  circle A205 centre (-7.5, -112.5) radius 1.7 projected
  circle A206 centre (-7.5, -117.5) radius 1.7 projected
  circle A207 centre (-7.5, -122.5) radius 1.7 projected
  circle A208 centre (-7.5, -127.5) radius 1.7 projected
  circle A209 centre (-7.5, -132.5) radius 1.7 projected
  circle A210 centre (-7.5, -137.5) radius 1.7 projected
  circle A211 centre (-7.5, -142.5) radius 1.7 projected
  circle A212 centre (-7.5, -147.5) radius 1.7 projected
  circle A213 centre (-7.5, -152.5) radius 1.7 projected
  circle A214 centre (-7.5, -157.5) radius 1.7 projected
  circle A215 centre (-7.5, -162.5) radius 1.7 projected
  circle A216 centre (-7.5, -167.5) radius 1.7 projected
  circle A217 centre (-7.5, -172.5) radius 1.7 projected
  circle A218 centre (-7.5, -177.5) radius 1.7 projected
  circle A219 centre (-7.5, -182.5) radius 1.7 projected
  circle A220 centre (-7.5, -187.5) radius 1.7 projected
  circle A221 centre (-7.5, -192.5) radius 1.7 projected
  circle A222 centre (-7.5, -197.5) radius 1.7 projected
  circle A223 centre (-7.5, -202.5) radius 1.7 projected
  circle A224 centre (-7.5, -207.5) radius 1.7 projected
  circle A225 centre (-7.5, -212.5) radius 1.7 projected
  circle A226 centre (-7.5, -217.5) radius 1.7 projected
  circle A227 centre (-7.5, -222.5) radius 1.7 projected
  circle A228 centre (-7.5, -227.5) radius 1.7 projected
  circle A229 centre (-7.5, -232.5) radius 1.7 projected
  circle A230 centre (-7.5, -237.5) radius 1.7 projected
  circle A231 centre (-7.5, -242.5) radius 1.7 projected
  circle A232 centre (-7.5, -247.5) radius 1.7 projected
  circle A233 centre (-7.5, -252.5) radius 1.7 projected
  circle A234 centre (-7.5, -257.5) radius 1.7 projected
  circle A235 centre (-7.5, -262.5) radius 1.7 projected
  circle A236 centre (-7.5, -267.5) radius 1.7 projected
  circle A237 centre (-7.5, -272.5) radius 1.7 projected
  circle A238 centre (-7.5, -277.5) radius 1.7 projected
  circle A239 centre (-7.5, -282.5) radius 1.7 projected
  circle A240 centre (-7.5, -287.5) radius 1.7 projected
  circle A241 centre (-7.5, -292.5) radius 1.7 projected
  circle A242 centre (-7.5, -297.5) radius 1.7 projected
  circle A243 centre (-7.5, -302.5) radius 1.7 projected
  circle A244 centre (2.5, -2.5) radius 1.7 projected
  circle A245 centre (2.5, -2.5) radius 1.7
  point P0 (0, 0)
  constraints: 1 centre point, 1 coincident
extrude "擠出8" add sketch "草圖7" along normal blind 1.5 contours A244
pattern_linear "矩形陣列6" count 61 spacing 5 along (0, 0, -1) of "擠出7", "擠出8"
